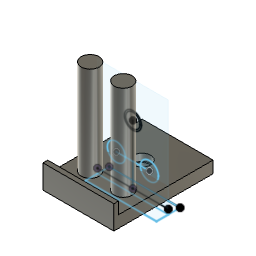
Lens_Holder (Autodesk Fusion 360 design; units mm, degrees)
Autodesk Fusion 360 part; units mm, degrees
sketch "Sketch1" plane through (0, 0, 0) normal (0, 0, 1) x (1, 0, 0)
  line L0 (-38.9102, 16.6955) -> (-8.9102, 16.6955)
  line L1 (-8.9102, 16.6955) -> (-8.9102, 6.6955)
  line L2 (-8.9102, 6.6955) -> (-38.9102, 6.6955)
  line L3 (-38.9102, 6.6955) -> (-38.9102, 16.6955)
  line L4 (-38.9102, 6.6955) -> (-8.9102, 6.6955)
  line L5 (-8.9102, 6.6955) -> (-8.9102, 11.6955)
  line L6 (-8.9102, 11.6955) -> (-38.9102, 11.6955)
  line L7 (-38.9102, 11.6955) -> (-38.9102, 6.6955)
  dimension "d1" = 30
  dimension "d2" = 10
  dimension "d3" = 5
  constraint horizontal L0
  constraint vertical L1
  constraint horizontal L2
  constraint vertical L3
  constraint horizontal L4
  constraint vertical L5
  constraint horizontal L6
  constraint vertical L7
  measures "d1" distance of L0.start L0.end
  measures "d2" distance of L0.start L2.end
  measures "d3" distance of L2.end L6.end
extrude "Extrude1" add sketch "Sketch1" along normal blind 42 contours L0 L1 L3 L6 makes body 1
extrude "Extrude2" add sketch "Sketch1" along normal blind 2 contours L1 L2 L3 L4 L5 L6 L7 bodies 1
sketch "Sketch2" plane through (0, 0, 0) normal (0, 1, 0) x (1, 0, 0)
  line L0 (-38.9102, 0, 16.6955) -> (-8.9102, 0, 16.6955)
  line L1 (-38.9102, -2, 11.6955) -> (-8.9102, -2, 11.6955)
  line L2 (-23.9102, -2, 11.6955) -> (-23.9102, -12, 11.6955)
  line L3 (-23.9102, -12, 11.6955) -> (-30.9102, -12, 11.6955)
  line L4 (-23.9102, -12, 11.6955) -> (-16.9102, -12, 11.6955)
  circle A0 through (-27.1102, -12, 11.6955) (-32.8102, -8.7091, 11.6955) (-32.8102, -15.2909, 11.6955)
  circle A1 through (-13.1102, -12, 11.6955) (-18.8102, -8.7091, 11.6955) (-18.8102, -15.2909, 11.6955)
  point P0 (-38.9102, 0)
  point P1 (-8.9102, 0)
  point P2 (-38.9102, -2)
  point P3 (-8.9102, -2)
  dimension "d11" = 10
  dimension "d12" = 7
  dimension "d13" = 7
  dimension "d14" = 7.6
  dimension "d15" = 7.6
extrude "Extrude3" add sketch "Sketch2" against normal blind 40 contours A0 in plane through (0, 11.6955, 0) normal (0, 1, 0) bodies 1
extrude "Extrude4" add sketch "Sketch2" against normal blind 40 contours A1 in plane through (0, 11.6955, 0) normal (0, 1, 0) bodies 1
sketch "Sketch3" plane through (0, 11.6955, 0) normal (0, -1, 0) x (1, 0, 0)
  circle A0 centre (-16.9102, 12) radius 3.8
  circle A1 centre (-30.9102, 12) radius 3.8
  line L0 (-38.9102, 2) -> (-8.9102, 2)
  line L1 (-8.9102, 2) -> (-8.9102, 42)
  line L2 (-8.9102, 42) -> (-38.9102, 42)
  line L3 (-38.9102, 42) -> (-38.9102, 2)
  line L4 (-23.9102, 2) -> (-23.9102, 27)
  circle A2 centre (-23.9102, 27) radius 3.6
  circle A3 centre (-23.9102, 27) radius 3
  point P0 (-23.9102, 2)
  dimension "d20" = 25
  dimension "d21" = 7.2
  dimension "d22" = 6
  constraint coincident P0 L4.start
  constraint perpendicular L0 L4
  constraint coincident L4.end A2.centre
  constraint concentric A2 A3
  measures "d20" distance of P0 L4.end
  measures "d21" diameter of A2
  measures "d22" diameter of A3
extrude "Extrude5" cut sketch "Sketch3" against normal blind 5 contours A3 bodies 1
extrude "Extrude6" cut sketch "Sketch3" against normal blind 3 contours A2 bodies 1
copy_body "Body->Comp1" bodies 1 removing the originals makes body 2 in component "Lens_Holder"
component "Lens_Holder" placed x (1, 0, 0) y (0, 1, 0) z (0, 0, 1) at (0, 0, 0)
